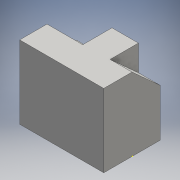
# Autodesk Inventor part: 240503_3Dsketch05
Saved by Autodesk Inventor 2016 (Build 200138000, 138)
## iProperties
Created: 2024-05-03
Part Number: 240503_3Dsketch05
Material: 일반
Document SubType Name: Modeling
Designer: pc
Density: 1 g/cm^3
Appearance: 기본값
Author: pc
Autodesk Inventor part; units mm, degrees
ref_plane "YZ Plane" through (0, 0, 0) normal (1, 0, 0) x (0, 1, 0)
ref_plane "XZ Plane" through (0, 0, 0) normal (0, 1, 0) x (-1, 0, 0)
ref_plane "XY Plane" through (0, 0, 0) normal (0, 0, 1) x (1, 0, 0)
sketch "스케치1" plane through (0, 0, 0) normal (0, 0, 1) x (1, 0, 0)
  line L0 (28.7473, -19.3425) -> (-28.7473, -19.3425)
  line L1 (-28.7473, -19.3425) -> (-28.7473, 19.3425)
  line L2 (-28.7473, 19.3425) -> (28.7473, 19.3425)
  line L3 (28.7473, 19.3425) -> (28.7473, -19.3425)
  line L4 (28.7473, -19.3425) -> (-28.7473, 19.3425) construction
  line L5 (-28.7473, -19.3425) -> (28.7473, 19.3425) construction
  point P0 (0, 0)
  constraints: 12 end point, 2 midpoint, 2 parallel, 1 horizontal, 1 perpendicular
extrude "돌출1" add sketch "스케치1" along normal blind 50
sketch "스케치2" plane through (-28.7473, 19.3425, 0) normal (0, 1, 0) x (1, 0, 0)
  line L0 (0, -50) -> (57.4945, -50) projected
  line L1 (0, -50) -> (24.4372, -50)
  line L2 (24.4372, -50) -> (24.4372, -30.5624)
  line L3 (24.4372, -30.5624) -> (0, -30.5624)
  line L4 (0, -30.5624) -> (0, -50)
  point P0 (28.7473, 0)
  constraints: 8 end point, 2 parallel, 1 horizontal, 1 perpendicular
extrude "돌출2" cut sketch "스케치2" against normal blind 20
sketch "스케치3" plane through (28.7473, -19.3425, 0) normal (1, 0, 0) x (0, 0, -1)
  point P0 (0, 19.3425)
sketch "스케치4" plane through (28.7473, -19.3425, 0) normal (1, 0, 0) x (0, 0, -1)
  line L0 (0, 38.685) -> (-50, 38.685) projected
  line L1 (-32.4307, 38.685) -> (-50, 19.3425)
  line L2 (-50, 0) -> (-50, 38.685) projected
  point P0 (0, 19.3425)
  constraints: 2 end point, 1 midpoint, 1 point on line
extrude "돌출3" cut sketch "스케치4" against normal blind 15
